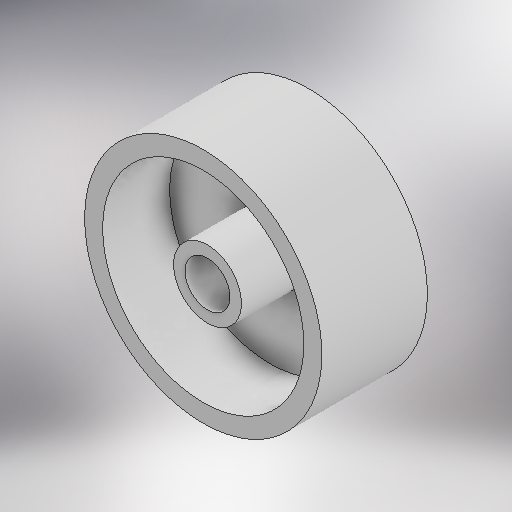
# Autodesk Inventor part: roda
Saved by Autodesk Inventor 2025.3 (Build 293356000, 356)
## iProperties
Created: 2026-09-16
Part Number: roda
Material: Genérico
Document SubType Name: Modeling
Designer: user
Density: 1 g/cm^3
Appearance: Padrão
Author: user
Autodesk Inventor part; units mm, degrees
ref_plane "YZ Plane" through (0, 0, 0) normal (1, 0, 0) x (0, 1, 0)
ref_plane "XZ Plane" through (0, 0, 0) normal (0, 1, 0) x (-1, 0, 0)
ref_plane "XY Plane" through (0, 0, 0) normal (0, 0, 1) x (1, 0, 0)
sketch "Esboço1" plane through (0, 0, 0) normal (0, 0, 1) x (1, 0, 0)
  circle A0 centre (0, 0) radius 16.8
  dimension "d0" = 33.6
  constraints: 1 centre point, 1 coincident
  measures "d0" diameter of A0
extrude "Extrusão1" add sketch "Esboço1" along normal blind 14.95
sketch "Esboço6" plane through (0, 0, 0) normal (0, 0, -1) x (-1, 0, 0)
  circle A0 centre (0, 0) radius 14.25
  dimension "d15" = 28.5
  constraints: 1 centre point, 1 coincident
  measures "d15" diameter of A0
extrude "Extrusão6" cut sketch "Esboço6" against normal blind 2.5
sketch "Esboço7" plane through (0, 0, 14.95) normal (0, 0, 1) x (1, 0, 0)
  circle A0 centre (0, 0) radius 14.25
  circle A1 centre (0, 0) radius 4.8
  dimension "d18" = 28.5
  dimension "d19" = 9.6
  constraints: 2 centre point, 2 coincident
  measures "d18" diameter of A0
  measures "d19" diameter of A1
extrude "Extrusão7" cut sketch "Esboço7" against normal blind 9.5
sketch "Esboço8" plane through (0, 0, 14.95) normal (0, 0, 1) x (1, 0, 0)
  circle A0 centre (0, 0) radius 4.8
  constraints: 1 centre point, 1 coincident
extrude "Extrusão8" cut sketch "Esboço8" against normal blind 0.6
sketch "Esboço9" plane through (0, 0, 14.35) normal (0, 0, 1) x (1, 0, 0)
  circle A0 centre (0, 0) radius 4.8 projected
  circle A1 centre (0, 0) radius 3.175
  dimension "d24" = 6.35
  constraints: 1 centre point, 1 coincident
  measures "d24" diameter of A1
extrude "Extrusão9" cut sketch "Esboço9" against normal blind 7.9 contours A1
sketch "Esboço10" plane through (0, 0, 6.45) normal (0, 0, 1) x (1, 0, 0)
  circle A0 centre (0, 0) radius 1.175
  dimension "d27" = 2.35
  constraints: 1 centre point, 1 coincident
  measures "d27" diameter of A0
extrude "Extrusão10" cut sketch "Esboço10" against normal blind 1.75
chamfer "Chanfro1" distance 0.25 angle 45 1 edges at (-1.175, 0, 6.45)
